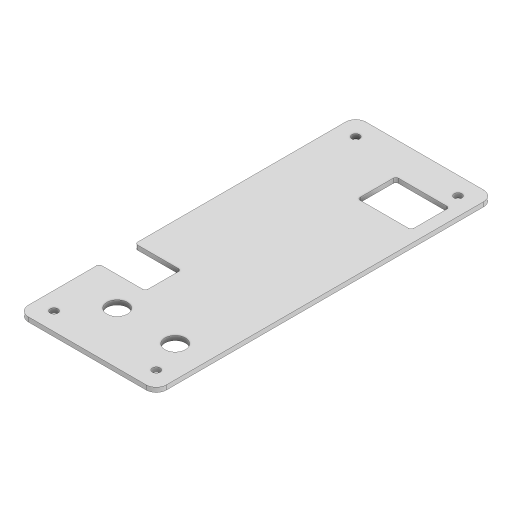
# Autodesk Inventor part: Control_PCB_enclosure_lid
Saved by Autodesk Inventor 2023 (Build 270158000, 158)
## iProperties
Created: 2026-04-14
Part Number: Control_PCB_enclosure_lid
Material: Generic
Document SubType Name: Modeling
Designer: ferrerx
Density: 1 g/cm^3
Appearance: Default
Author: ferrerx
Autodesk Inventor part; units mm, degrees
ref_plane "YZ Plane" through (0, 0, 0) normal (1, 0, 0) x (0, 1, 0)
ref_plane "XZ Plane" through (0, 0, 0) normal (0, 1, 0) x (-1, 0, 0)
ref_plane "XY Plane" through (0, 0, 0) normal (0, 0, 1) x (1, 0, 0)
sketch "Sketch1" plane through (0, 0, 0) normal (0, 1, 0) x (-1, 0, 0)
  line L0 (-24, 63) -> (24, 63)
  line L1 (24, 63) -> (24, -63)
  line L2 (24, -63) -> (-24, -63)
  line L3 (-24, -63) -> (-24, 63)
  line L4 (-24, 63) -> (24, -63) construction
  line L5 (24, 63) -> (-24, -63) construction
  line L6 (-20, 59) -> (20, 59) construction
  line L7 (20, 59) -> (20, -59) construction
  line L8 (20, -59) -> (-20, -59) construction
  line L9 (-20, -59) -> (-20, 59) construction
  line L10 (-20, 59) -> (20, -59) construction
  line L11 (20, 59) -> (-20, -59) construction
  circle A0 centre (20, 59) radius 1.55
  circle A1 centre (20, -59) radius 1.55
  circle A2 centre (-20, -59) radius 1.55
  circle A3 centre (-20, 59) radius 1.55
  point P0 (0, 0)
  dimension "d0" = 126
  dimension "d1" = 48
  dimension "d2" = 3.1
  dimension "d3" = 4
  dimension "d4" = 4
  dimension "d5" = 3.1
  dimension "d6" = 3.1
  dimension "d7" = 3.1
  constraints: 24 end point, 4 centre point, 4 coincident, 4 midpoint, 4 parallel, 2 horizontal, 2 perpendicular
  measures "d0" distance of L0.end L1.end
  measures "d1" distance of L0.start L0.end
  measures "d2" diameter of A0
  measures "d3" distance between parallel lines of L1 L7
  measures "d4" distance between parallel lines of L0 L6
  measures "d5" diameter of A3
  measures "d6" diameter of A2
  measures "d7" diameter of A1
extrude "Extrusion1" add sketch "Sketch1" along normal blind 1.6
fillet "Fillet1" radius 5 4 edges at (24, 0.8, -63) (-24, 0.8, -63) (24, 0.8, 63) (-24, 0.8, 63)
sketch "Sketch2" plane through (0, 0, 0) normal (0, -1, 0) x (1, 0, 0)
  circle A0 centre (20, 59) radius 1.55 projected
  circle A1 centre (20, 59) radius 2.1
  circle A2 centre (20, 59) radius 3.5
  line L0 (0, 0) -> (23.8307, 0) construction
  line L1 (0, 0) -> (0, 62.8307) construction
  circle A3 centre (20, -59) radius 1.55
  circle A4 centre (20, -59) radius 2.1
  circle A5 centre (20, -59) radius 3.5
  circle A6 centre (-20, 59) radius 1.55
  circle A7 centre (-20, 59) radius 2.1
  circle A8 centre (-20, 59) radius 3.5
  circle A9 centre (-20, -59) radius 1.55
  circle A10 centre (-20, -59) radius 2.1
  circle A11 centre (-20, -59) radius 3.5
  point P0 (-23.8307, 0)
  dimension "d11" = 4.2
  dimension "d12" = 7
  constraints: 11 centre point, 11 symmetric about line, 8 coincident, 4 end point, 1 horizontal, 1 vertical, 9 other
  measures "d11" diameter of A1
  measures "d12" diameter of A2
extrude "Extrusion2" add sketch "Sketch2" along normal blind 6.5 contours A2 | A5 | A8 | A11
sketch "Sketch3" plane through (20, -6.5, -59) normal (0, -1, 0) x (1, 0, 0)
  line L0 (-47, 125) -> (7, 125)
  line L1 (7, 125) -> (7, -7)
  line L2 (7, -7) -> (-47, -7)
  line L3 (-47, -7) -> (-47, 125)
  line L4 (-47, 125) -> (7, -7) construction
  line L5 (7, 125) -> (-47, -7) construction
  line L6 (4, 117) -> (4, 1) projected
  line L7 (-39, 122) -> (-1, 122) projected
  point P0 (-20, 59)
  dimension "d17" = 3
  dimension "d18" = 3
  constraints: 12 end point, 2 midpoint, 2 parallel, 1 horizontal, 1 perpendicular
  measures "d17" distance between parallel lines of L6 L1
  measures "d18" distance between parallel lines of L0 L7
extrude "Extrusion3" add sketch "Sketch3" along normal blind 2
sketch "Sketch4" plane through (20, -6.5, -59) normal (0, 1, 0) x (1, 0, 0)
  line L0 (-47, 7) -> (7, 7) projected
  line L1 (7, -125) -> (-47, -125)
  line L2 (-47, -125) -> (-47, 7)
  line L3 (-47, 7) -> (7, 7)
  line L4 (7, 7) -> (7, -125)
  line L5 (7, -125) -> (-47, 7) construction
  line L6 (-47, -125) -> (7, 7) construction
  line L7 (5, -123) -> (-45, -123)
  line L8 (-45, -123) -> (-45, 5)
  line L9 (-45, 5) -> (5, 5)
  line L10 (5, 5) -> (5, -123)
  line L11 (5, -123) -> (-45, 5) construction
  line L12 (-45, -123) -> (5, 5) construction
  point P0 (-20, -59)
  dimension "d21" = 2
  dimension "d22" = 2
  constraints: 24 end point, 4 midpoint, 4 parallel, 2 horizontal, 2 perpendicular
  measures "d21" distance between parallel lines of L0 L9
  measures "d22" distance between parallel lines of L2 L8
extrude "Extrusion4" add sketch "Sketch4" along normal blind 24
sketch "Sketch5" plane through (-25, -6.5, 64) normal (1, 0, 0) x (0, 0, -1)
  circle A0 centre (110.2, 15.2) radius 4
  line L0 (6, 6.5) -> (122, 6.5) projected
  point P0 (64, 6.5)
  point P1 (1, 8.1)
  point P2 (127, 8.1)
  point P3 (108.5902, 6.5)
  point P4 (111.8098, 6.5)
  dimension "d25" = 8.7
  dimension "d27" = 16.8
  dimension "d28" = 8
  constraints: 1 centre point
  measures "d25" distance from line of L0 A0.centre
  measures "d27" horizontal distance of point (127, 8.1) A0.centre
  measures "d28" diameter of A0
extrude "Extrusion5" cut sketch "Sketch5" against normal blind 15.5
sketch "Sketch6" plane through (25, -6.5, -64) normal (-1, 0, 0) x (0, 0, 1)
  line L0 (28.9, 21.7) -> (44.6, 21.7)
  line L1 (44.6, 21.7) -> (44.6, 8.1)
  line L2 (44.6, 8.1) -> (28.9, 8.1)
  line L3 (28.9, 8.1) -> (28.9, 21.7)
  line L4 (122, 8.1) -> (6, 8.1) projected
  point P0 (64, 6.5)
  point P1 (1, 8.1)
  dimension "d31" = 43.6
  dimension "d32" = 15.7
  dimension "d33" = 13.6
  constraints: 8 end point, 2 parallel, 1 collinear, 1 horizontal, 1 perpendicular
  measures "d31" distance from line of point (1, 8.1) L1
  measures "d32" distance of L0.start L0.end
  measures "d33" distance of L0.end L1.end
extrude "Extrusion6" cut sketch "Sketch6" against normal blind 15.5
fillet "Fillet2" radius 1 4 edges at (26, 1.6, -35.1) (26, 1.6, -19.4) (26, 15.2, -19.4) (26, 15.2, -35.1)
sketch "Sketch7" plane through (-27, -8.5, -66) normal (-1, 0, 0) x (0, 0, 1)
  line L0 (86.3, 29.1) -> (100.3, 29.1)
  line L1 (100.3, 29.1) -> (100.3, 19.1)
  line L2 (100.3, 19.1) -> (86.3, 19.1)
  line L3 (86.3, 19.1) -> (86.3, 29.1)
  line L4 (86.3, 29.1) -> (100.3, 19.1) construction
  line L5 (100.3, 29.1) -> (86.3, 19.1) construction
  line L6 (8, 10.1) -> (124, 10.1) projected
  point P0 (66, 8.5)
  point P1 (93.3, 24.1)
  point P2 (129, 10.1)
  dimension "d37" = 14
  dimension "d38" = 10
  dimension "d39" = 35.7
  dimension "d40" = 14
  constraints: 12 end point, 2 midpoint, 2 parallel, 1 horizontal, 1 perpendicular
  measures "d37" distance of L0.start L0.end
  measures "d38" distance of L0.end L1.end
  measures "d39" horizontal distance of point (129, 10.1) point (93.3, 24.1)
  measures "d40" distance from line of L6 point (93.3, 24.1)
extrude "Extrusion7" cut sketch "Sketch7" against normal blind 15.5
sketch "Sketch8" plane through (0, 1.6, 0) normal (0, 1, 0) x (1, 0, 0)
  line L0 (-24, 63) -> (24, 63)
  line L1 (24, 63) -> (24, -63)
  line L2 (24, -63) -> (-24, -63)
  line L3 (-24, -63) -> (-24, 63)
  line L4 (-24, 63) -> (24, -63) construction
  line L5 (24, 63) -> (-24, -63) construction
  line L6 (24, -58) -> (24, 58) projected
  line L7 (19, 63) -> (-19, 63) projected
  point P0 (0, 0)
  constraints: 12 end point, 2 collinear, 2 midpoint, 2 parallel, 1 horizontal, 1 perpendicular
extrude "Extrusion8" cut sketch "Sketch8" against normal blind 1.6
fillet "Fillet4" radius 3 4 edges at (25, 5.5, -64) (25, 5.5, 64) (-25, 5.5, 64) (-25, 5.5, -64)
fillet "Fillet5" radius 4 4 edges at (-27, 4.5, 66) (-27, 4.5, -66) (27, 4.5, -66) (27, 4.5, 66)
sketch "Sketch9" plane through (20, 17.5, -59) normal (0, 1, 0) x (1, 0, 0)
  line L0 (-47, -79.3) -> (-45, -79.3) projected
  line L1 (-47, -79.3) -> (-29, -79.3)
  line L2 (-29, -79.3) -> (-29, -93.3)
  line L3 (-29, -93.3) -> (-47, -93.3)
  line L4 (-47, -93.3) -> (-47, -79.3)
  line L5 (-45, -93.3) -> (-47, -93.3) projected
  point P0 (-20, -59)
  dimension "d48" = 18
  constraints: 8 end point, 2 parallel, 1 collinear, 1 horizontal, 1 perpendicular
  measures "d48" distance of L2.end L3.end
extrude "Extrusion9" cut sketch "Sketch9" against normal blind 26.5
sketch "Sketch10" plane through (20, -6.5, -59) normal (0, 1, 0) x (1, 0, 0)
  line L0 (2.35, -5.66) -> (-18.65, -5.66)
  line L1 (-18.65, -5.66) -> (-18.65, -20.66)
  line L2 (-18.65, -20.66) -> (2.35, -20.66)
  line L3 (2.35, -20.66) -> (2.35, -5.66)
  line L4 (3, 7) -> (-43, 7) projected
  line L5 (7, -121) -> (7, 3) projected
  point P0 (-20, -59)
  dimension "d51" = 27.66
  dimension "d52" = 21
  dimension "d53" = 15
  dimension "d54" = 25.65
  constraints: 8 end point, 2 parallel, 1 horizontal, 1 perpendicular
  measures "d51" distance between parallel lines of L4 L2
  measures "d52" distance of L1.end L2.end
  measures "d53" distance of L0.end L1.end
  measures "d54" distance between parallel lines of L5 L1
extrude "Extrusion10" cut sketch "Sketch10" against normal blind 26.5
fillet "Fillet6" radius 1 4 edges at (22.35, -7.5, -53.34) (22.35, -7.5, -38.34) (1.35, -7.5, -38.34) (1.35, -7.5, -53.34)
sketch "Sketch11" plane through (20, -6.5, -59) normal (0, 1, 0) x (1, 0, 0)
  circle A0 centre (-5.2, -105.4) radius 4
  circle A1 centre (-28.6, -104.7) radius 4
  line L0 (-43, -125) -> (3, -125) projected
  line L1 (7, -121) -> (7, 3) projected
  line L2 (-47, -93.3) -> (-47, -121) projected
  point P0 (-20, -59)
  dimension "d58" = 19.6
  dimension "d59" = 12.2
  dimension "d60" = 8
  dimension "d61" = 20.3
  dimension "d62" = 18.4
  dimension "d63" = 8
  constraints: 2 centre point
  measures "d58" distance from line of L0 A0.centre
  measures "d59" distance from line of L1 A0.centre
  measures "d60" diameter of A0
  measures "d61" distance from line of L0 A1.centre
  measures "d62" distance from line of L2 A1.centre
  measures "d63" diameter of A1
extrude "Extrusion11" cut sketch "Sketch11" against normal blind 26.5
sketch "Sketch13" plane through (20, -6.5, 59) normal (0, 1, 0) x (1, 0, 0)
  circle A0 centre (0, 0) radius 1.5
  circle A1 centre (0, 118) radius 2.1 projected
  circle A2 centre (0, 118) radius 1.5
  circle A3 centre (-40, 118) radius 2.1 projected
  circle A4 centre (-40, 118) radius 1.5
  circle A5 centre (-40, 0) radius 2.1 projected
  circle A6 centre (-40, 0) radius 1.5
  point P0 (-20, 59)
  dimension "d69" = 3
  dimension "d70" = 3
  dimension "d71" = 3
  dimension "d72" = 3
  constraints: 4 centre point, 3 coincident
  measures "d69" diameter of A0
  measures "d70" diameter of A2
  measures "d71" diameter of A4
  measures "d72" diameter of A6
extrude "Extrusion13" cut sketch "Sketch13" against normal blind 24.25 contours A0 | A2 | A4 | A6
sketch "Sketch12" plane through (20, 17.5, -59) normal (0, 1, 0) x (1, 0, 0)
  line L0 (-55.8435, 27.803) -> (15.8435, 27.803)
  line L1 (15.8435, 27.803) -> (15.8435, -145.803)
  line L2 (15.8435, -145.803) -> (-55.8435, -145.803)
  line L3 (-55.8435, -145.803) -> (-55.8435, 27.803)
  line L4 (-55.8435, 27.803) -> (15.8435, -145.803) construction
  line L5 (15.8435, 27.803) -> (-55.8435, -145.803) construction
  point P0 (-20, -59)
  constraints: 12 end point, 2 midpoint, 2 parallel, 1 horizontal, 1 perpendicular
extrude "Extrusion12" cut sketch "Sketch12" against normal blind 24.25
fillet "Fillet7" radius 1 4 edges at (-9, -7.625, 20.3) (-9, -7.625, 34.3) (-27, -7.625, 20.3) (-27, -7.625, 34.3)
equation "\"d5\" = d2"
equation "\"d6\" = d2"
equation "\"d7\" = d2"
equation "\"d63\" = d60"
body "Solid1"
